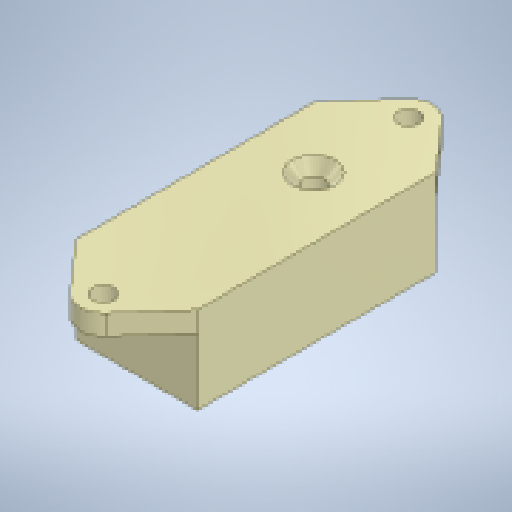
# Autodesk Inventor part: креп_опт
Saved by Autodesk Inventor 2023.1 (Build 271208000, 208)
## iProperties
Created: 2025-12-30
Part Number: креп_опт
Material: Полипропилен
Document SubType Name: Modeling
Designer: DELL
Density: 0.899 g/cm^3
Appearance: Гладкий — пепельный
Author: DELL
Autodesk Inventor part; units mm, degrees
ref_plane "YZ Plane" through (0, 0, 0) normal (1, 0, 0) x (0, 1, 0)
ref_plane "XZ Plane" through (0, 0, 0) normal (0, 1, 0) x (-1, 0, 0)
ref_plane "XY Plane" through (0, 0, 0) normal (0, 0, 1) x (1, 0, 0)
sketch "Эскиз1" plane through (0, 0, 0) normal (0, 1, 0) x (-1, 0, 0)
  line L0 (7.1, -15.85) -> (-7.1, -15.85)
  line L1 (-7.1, -15.85) -> (-7.1, 15.85)
  line L2 (-7.1, 15.85) -> (7.1, 15.85)
  line L3 (7.1, 15.85) -> (7.1, -15.85)
  line L4 (7.1, -15.85) -> (-7.1, 15.85) construction
  line L5 (-7.1, -15.85) -> (7.1, 15.85) construction
  line L6 (9.1, -17.85) -> (-9.1, -17.85)
  line L7 (-9.1, -17.85) -> (-9.1, 17.85)
  line L8 (-9.1, 17.85) -> (9.1, 17.85)
  line L9 (9.1, 17.85) -> (9.1, -17.85)
  point P0 (0, 0)
  dimension "d0" = 14.2
  dimension "d1" = 31.7
  dimension "d2" = 2
  constraints: 20 end point, 4 parallel, 2 midpoint, 2 perpendicular, 1 horizontal, 3 other
  measures "d0" distance of L1.end L2.end
  measures "d1" distance of L2.end L0.start
  measures "d2" distance between parallel lines of L3 L9
extrude "Выдавливание1" add sketch "Эскиз1" along normal blind 10
sketch "Эскиз2" plane through (0, 10, 0) normal (0, 1, 0) x (1, 0, 0)
  line L0 (-9.1, 17.85) -> (-9.1, -17.85) projected
  line L1 (-9.1, -17.85) -> (9.1, -17.85) projected
  line L2 (9.1, -17.85) -> (9.1, 17.85) projected
  line L3 (9.1, 17.85) -> (-9.1, 17.85) projected
  point P0 (0, 0)
extrude "Выдавливание2" add sketch "Эскиз2" along normal blind 3
sketch "Эскиз4" plane through (9.1, 0, -17.85) normal (0, 0, -1) x (-1, 0, 0)
  line L0 (0, 0) -> (0, 13) construction
  line L1 (0, 0) -> (0, 13) construction
  line L2 (0, 0) -> (18.2, 0) construction
  line L3 (18.2, 0) -> (18.2, 13) construction
  line L4 (18.2, 0) -> (18.2, 13) construction
  line L5 (0, 0) -> (0, 13) projected
  line L6 (0, 0) -> (0, 13)
  line L7 (18.2, 0) -> (0, 0) projected
  line L8 (0, 0) -> (18.2, 0)
  line L9 (18.2, 0) -> (18.2, 13)
  line L10 (5.972, 13) -> (0, 13)
  line L11 (0, 13) -> (18.2, 13)
  line L12 (0, 0) -> (0, 13) projected
  line L13 (0, 13) -> (0, 7)
  line L14 (2, 0) -> (2, 10)
  line L15 (2, 10) -> (16.2, 10)
  line L16 (16.2, 10) -> (16.2, 0)
  point P0 (9.1, 0)
  point P1 (18.2, 7)
  point P2 (0, 6.5)
  point P3 (18.2, 6.5)
  point P4 (16.2, 0)
  dimension "d0" = 14.2
  dimension "d15" = 2
  dimension "d16" = 2
  dimension "d53" = 10
  constraints: 18 end point, 4 perpendicular, 3 collinear, 2 midpoint, 2 point on line
  measures "d15" distance from line of point (0, 6.5) L14
  measures "d16" distance from line of point (18.2, 6.5) L16
  measures "d53" distance between parallel lines of L15 L2
extrude "Выдавливание4" cut sketch "Эскиз4" against normal blind 3 contours L14 L15 L16 L7
sketch "Эскиз5" plane through (0, 13, 0) normal (0, 1, 0) x (1, 0, 0)
  line L0 (0, 0) -> (0, -28.4562) construction
  circle A0 centre (0, -22.85) radius 1.6
  circle A1 centre (0, 22.85) radius 1.6
  line L1 (-9.1, -17.85) -> (9.1, -17.85) projected
  line L2 (9.1, 17.85) -> (-9.1, 17.85) projected
  arc A2 (2.6208, 25.1698) -> (-2.6208, 25.1698) centre (0, 22.85) ccw
  arc A3 (-2.6208, -25.1698) -> (2.6208, -25.1698) centre (0, -22.85) ccw
  line L3 (9.1, 17.85) -> (-9.1, 17.85) projected
  line L4 (9.1, 17.85) -> (2.6208, 25.1698)
  line L5 (-9.1, 17.85) -> (-2.6208, 25.1698)
  line L6 (-9.1, -17.85) -> (-2.6208, -25.1698)
  line L7 (9.1, -17.85) -> (9.1, 17.85) projected
  line L8 (9.1, -17.85) -> (2.6208, -25.1698)
  point P0 (7.1, 17.85)
  dimension "d32" = 3.2
  dimension "d33" = 3.2
  dimension "d34" = 5
  dimension "d35" = 5
  dimension "d36" = 7
  dimension "d37" = 7
  constraints: 10 end point, 4 centre point, 4 point on circle, 4 tangent, 2 coincident, 1 point on line, 1 vertical
  measures "d32" diameter of A0
  measures "d33" diameter of A1
  measures "d34" distance from line of L1 A0.centre
  measures "d35" distance from line of L2 A1.centre
  measures "d36" diameter of A2
  measures "d37" diameter of A3
extrude "Выдавливание5" add sketch "Эскиз5" against normal blind 3
sketch "Эскиз6" plane through (0, 10, 0) normal (0, -1, 0) x (1, 0, 0)
  circle A0 centre (0, -8.65) radius 1.5 construction
  circle A1 centre (0, -8.65) radius 1.6
  point P0 (0, 0)
  dimension "d38" = 3.2
  constraints: 1 centre point, 1 coincident
  measures "d38" diameter of A1
extrude "Выдавливание6" cut sketch "Эскиз6" against normal blind 10
chamfer "Фаска1" distance 1.65 angle 45 1 edges at (-1.6, 13, -8.65)
sketch "Эскиз7" plane through (0, 10, 0) normal (0, -1, 0) x (1, 0, 0)
  circle A0 centre (0, -8.65) radius 1.6 projected
  circle A1 centre (0, -8.65) radius 1.6
  circle A2 centre (0, -8.65) radius 2.5
  point P0 (0, 0)
  dimension "d44" = 5
  constraints: 2 centre point, 2 coincident
  measures "d44" diameter of A2
extrude "Выдавливание7" add sketch "Эскиз7" along normal blind 8.4
chamfer "Фаска3" distance 1 angle 45 1 edges at (-2.5, 10, -8.65)
